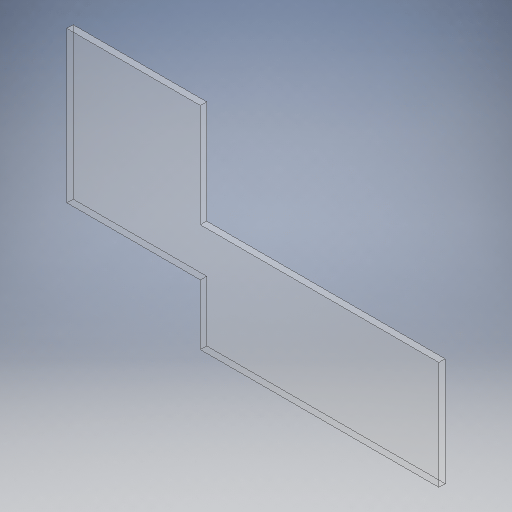
# Autodesk Inventor part: cowl_left
Saved by Autodesk Inventor 2025.2 (Build 292293000, 293)
## iProperties
Created: 2025-02-07
Part Number: cowl_left
Material: 폴리카보네이트, 선명
Document SubType Name: Modeling
Designer: jbhma
Density: 1.2 g/cm^3
Appearance: 폴리카보네이트 - 선명
Author: jbhma
Autodesk Inventor part; units mm, degrees
ref_plane "YZ Plane" through (0, 0, 0) normal (1, 0, 0) x (0, 1, 0)
ref_plane "XZ Plane" through (0, 0, 0) normal (0, 1, 0) x (-1, 0, 0)
ref_plane "XY Plane" through (0, 0, 0) normal (0, 0, 1) x (1, 0, 0)
sketch "스케치2" plane through (0, 0, 0) normal (0, 0, 1) x (1, 0, 0)
  line L0 (0, 0) -> (420, 0)
  line L1 (420, 0) -> (420, -475)
  line L2 (420, -475) -> (0, -475)
  line L3 (0, -475) -> (0, 0)
  line L4 (420, -325) -> (1170, -325)
  line L5 (1170, -325) -> (1170, -665)
  line L6 (1170, -665) -> (420, -665)
  line L7 (420, -665) -> (420, -325)
  dimension "d6" = 420
  dimension "d7" = 475
  dimension "d8" = 750
  dimension "d9" = 340
  constraints: 16 end point, 4 parallel, 2 horizontal, 2 perpendicular, 1 point on line
  measures "d6" distance of L1.end L2.end
  measures "d7" distance of L0.end L1.end
  measures "d8" distance of L5.end L6.end
  measures "d9" distance of L4.end L5.end
extrude "돌출2" add sketch "스케치2" along normal blind 20
